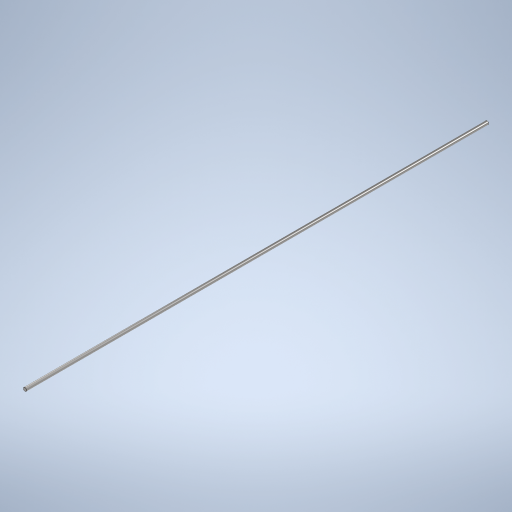
# Autodesk Inventor part: Linear Rod
Saved by Autodesk Inventor 2023 (Build 270158000, 158)
## iProperties
Created: 2023-02-13
Part Number: Linear Rod
Material: Stainless Steel
Document SubType Name: Modeling
Designer: mbear
Density: 8 g/cm^3
Appearance: Semi-Polished
Mass: 241.268 g
Surface Area: 201.534 cm^2
Volume: 30.1585 cm^3
Author: mbear
Autodesk Inventor part; units mm, degrees
ref_plane "YZ Plane" through (0, 0, 0) normal (1, 0, 0) x (0, 1, 0)
ref_plane "XZ Plane" through (0, 0, 0) normal (0, 1, 0) x (-1, 0, 0)
ref_plane "XY Plane" through (0, 0, 0) normal (0, 0, 1) x (1, 0, 0)
sketch "Sketch1" plane through (0, 0, 0) normal (0, 0, 1) x (1, 0, 0)
  circle A0 centre (0, 0) radius 4
  dimension "d0" = 8
  constraints: 1 centre point, 1 coincident
  measures "d0" diameter of A0
extrude "Extrusion1" add sketch "Sketch1" along normal blind 1066.8
chamfer "Chamfer1" distance 0.508 angle 45 2 edges at (-4, 0, 0) (-4, 0, 1066.8)
body "Solid1"
